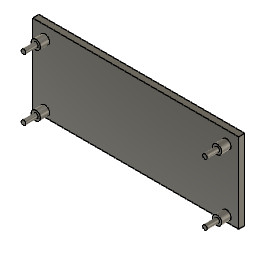
pb2-1 v3 (Autodesk Fusion 360 design; units mm, degrees)
Autodesk Fusion 360 part; units mm, degrees
sketch "Sketch1" plane through (0, 0, 0) normal (0, 1, 0) x (1, 0, 0)
  line L0 (0, 0) -> (67, 0)
  line L1 (67, 0) -> (67, -26)
  line L2 (67, -26) -> (0, -26)
  line L3 (0, -26) -> (0, 0)
  dimension "d1" = 67
  dimension "d2" = 26
  constraint horizontal L0
  constraint vertical L1
  constraint horizontal L2
  constraint vertical L3
  constraint coincident L0.start L3.end
  measures "d1" distance of L1.end L2.end
  measures "d2" distance of L0.start L2.end
extrude "Extrude1" add sketch "Sketch1" along normal blind 2
sketch "Sketch2" plane through (0, 0, 0) normal (0, 1, 0) x (1, 0, 0)
  circle A0 centre (4, -2) radius 1.5
  circle A1 centre (63, -2) radius 1.5
  circle A2 centre (4, -22) radius 1.5
  circle A3 centre (63, -22) radius 1.5
  dimension "d5" = 3
  dimension "d6" = 3
  dimension "d7" = 3
  dimension "d8" = 3
  measures "d5" diameter of A0
  measures "d6" diameter of A1
  measures "d7" diameter of A2
  measures "d8" diameter of A3
extrude "Extrude2" add sketch "Sketch2" against normal blind 3
sketch "Sketch3" plane through (0, 0, 0) normal (0, 1, 0) x (1, 0, 0)
  circle A0 centre (4, -22) radius 0.75
  circle A1 centre (4, -2) radius 0.75
  circle A2 centre (63, -22) radius 0.75
  circle A3 centre (63, -2) radius 0.75
  dimension "d11" = 1.5
  dimension "d12" = 1.5
  dimension "d13" = 1.5
  dimension "d14" = 1.5
  measures "d11" diameter of A0
  measures "d12" diameter of A1
  measures "d13" diameter of A2
  measures "d14" diameter of A3
extrude "Extrude3" add sketch "Sketch3" against normal blind 7 contours A0
sketch "Sketch4" plane through (0, 0, 0) normal (0, 1, 0) x (1, 0, 0)
  circle A0 centre (4, -2) radius 0.75
  dimension "d17" = 1.5
  measures "d17" diameter of A0
extrude "Extrude4" add sketch "Sketch4" against normal blind 7
sketch "Sketch5" plane through (0, 0, 0) normal (0, 1, 0) x (1, 0, 0)
  circle A0 centre (63, -22) radius 0.75
  dimension "d20" = 1.5
  measures "d20" diameter of A0
extrude "Extrude5" add sketch "Sketch5" against normal blind 7
sketch "Sketch6" plane through (0, 0, 0) normal (0, 1, 0) x (1, 0, 0)
  circle A0 centre (63, -2) radius 0.75
  dimension "d23" = 1.5
  measures "d23" diameter of A0
extrude "Extrude6" add sketch "Sketch6" against normal blind 7
